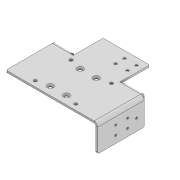
# Autodesk Inventor part: CCM_Mount_G
Saved by Autodesk Inventor 2020 (Build 240168000, 168)
## iProperties
Created: 2021-07-12
Part Number: CCM_Mount_G
Material: 一般
Document SubType Name: Sheet Metal
Designer: magnarecta
Density: 1 g/cm^3
Appearance: 既定
Sheet Metal Rule: Default
Author: magnarecta
Autodesk Inventor part; units mm, degrees
ref_plane "YZ Plane" through (0, 0, 0) normal (1, 0, 0) x (0, 1, 0)
ref_plane "XZ Plane" through (0, 0, 0) normal (0, 1, 0) x (-1, 0, 0)
ref_plane "XY Plane" through (0, 0, 0) normal (0, 0, 1) x (1, 0, 0)
sketch "スケッチ1" plane through (0, 0, 0) normal (0, 1, 0) x (-1, 0, 0)
  line L0 (-40, -39) -> (40, -39)
  line L1 (40, -39) -> (40, 39)
  line L2 (40, 39) -> (-40, 39)
  line L3 (-40, 39) -> (-40, -39)
  line L4 (-40, -39) -> (40, 39) construction
  line L5 (40, -39) -> (-40, 39) construction
  point P0 (0, 0)
  dimension "d0" = 80
  dimension "d1" = 78
  constraints: 12 end point, 2 midpoint, 2 parallel, 1 horizontal, 1 perpendicular
  measures "d0" distance of L0.start L0.end
  measures "d1" distance of L0.end L1.end
extrude "押し出し1" add sketch "スケッチ1" along normal blind 3
sketch "スケッチ2" plane through (0, 3, 0) normal (0, 1, 0) x (1, 0, 0)
  line L0 (34, 30) -> (-34, 30)
  line L1 (-34, 30) -> (-34, -30)
  line L2 (-34, -30) -> (34, -30)
  line L3 (34, -30) -> (34, 30)
  line L4 (34, 30) -> (-34, -30) construction
  line L5 (-34, 30) -> (34, -30) construction
  point P0 (0, 0)
  dimension "d4" = 68
  dimension "d5" = 60
  constraints: 12 end point, 2 midpoint, 2 parallel, 1 horizontal, 1 perpendicular
  measures "d4" distance of L2.end L1.end
  measures "d5" distance of L1.end L0.end
hole "穴1" at (-34, 3, 30) at (34, 3, 30) at (34, 3, -30) at (-34, 3, -30) direction (0, -1, 0) diameter 5.2 depth 8 tip angle 118
sketch "スケッチ3" plane through (0, 3, 0) normal (0, 1, 0) x (1, 0, 0)
  line L0 (13.5, 25) -> (-13.5, 25)
  line L1 (-13.5, 25) -> (-13.5, -25)
  line L2 (-13.5, -25) -> (13.5, -25)
  line L3 (13.5, -25) -> (13.5, 25)
  line L4 (13.5, 25) -> (-13.5, -25) construction
  line L5 (-13.5, 25) -> (13.5, -25) construction
  point P0 (0, 0)
  dimension "d13" = 27
  dimension "d14" = 50
  constraints: 12 end point, 4 coincident, 2 midpoint, 2 parallel, 1 horizontal, 1 perpendicular
  measures "d13" distance of L0.start L0.end
  measures "d14" distance of L0.end L1.end
hole "穴2" at (-13.5, 3, 25) at (13.5, 3, 25) at (13.5, 3, -25) at (-13.5, 3, -25) direction (0, -1, 0) diameter 5.3 depth 8 tip angle 118 countersink diameter 10 countersink angle 90
sketch "スケッチ5" plane through (0, 0, 0) normal (0, -1, 0) x (1, 0, 0)
  line L0 (74, 39) -> (-74, 39)
  line L1 (-74, 39) -> (-74, -39)
  line L2 (-74, -39) -> (74, -39)
  line L3 (74, -39) -> (74, 39)
  circle A0 centre (13.5, -25) radius 2.65 projected
  circle A1 centre (13.5, -25) radius 2.65 projected
  circle A2 centre (-13.5, 25) radius 2.65 projected
  circle A3 centre (13.5, 25) radius 2.65 projected
  circle A4 centre (-13.5, -25) radius 2.65 projected
  circle A5 centre (34, -30) radius 2.6 projected
  circle A6 centre (-34, 30) radius 2.6 projected
  circle A7 centre (34, 30) radius 2.6 projected
  circle A8 centre (-34, -30) radius 2.6 projected
  line L4 (-40, -39) -> (-40, 39) projected
  line L5 (40, -39) -> (-40, -39) projected
  line L6 (40, 39) -> (40, -39) projected
  line L7 (-40, 39) -> (40, 39) projected
  point P0 (0, 0)
  point P1 (-40, 39)
  dimension "d28" = 40
  dimension "d29" = 40
  constraints: 8 end point, 2 horizontal alignment, 2 parallel, 1 horizontal, 1 perpendicular
  measures "d28" distance from line of A5.centre L3
  measures "d29" distance from line of L1 A8.centre
extrude "押し出し3" add sketch "スケッチ5" against normal up to surface (3 mm away) contours L3 L2 L6 L0 | L4 L2 L1 L0
sketch "スケッチ6" plane through (0, 0, 0) normal (0, -1, 0) x (1, 0, 0)
  circle A0 centre (13.5, -25) radius 2.65 projected
  circle A1 centre (-13.5, 25) radius 2.65 projected
  circle A2 centre (13.5, 25) radius 2.65 projected
  circle A3 centre (-13.5, -25) radius 2.65 projected
  circle A4 centre (34, -30) radius 2.6 projected
  circle A5 centre (-34, 30) radius 2.6 projected
  circle A6 centre (34, 30) radius 2.6 projected
  circle A7 centre (-34, -30) radius 2.6 projected
  line L0 (-74, -39) -> (74, -39) projected
  line L1 (74, -39) -> (74, 39) projected
  line L2 (74, 39) -> (-74, 39) projected
  line L3 (-74, 39) -> (-74, -39) projected
  line L4 (74, -39) -> (44, -39)
  line L5 (44, -39) -> (44, -42)
  line L6 (44, -42) -> (74, -42)
  line L7 (74, -42) -> (74, -39)
  line L8 (-74, 39) -> (-74, -39) projected
  line L9 (-74, -39) -> (-44, -39)
  line L10 (-44, -39) -> (-44, -42)
  line L11 (-44, -42) -> (-74, -42)
  line L12 (-74, -42) -> (-74, -39)
  line L13 (44, -42) -> (-44, -42)
  line L14 (-44, -42) -> (-44, -39)
  line L15 (-44, -39) -> (44, -39)
  line L16 (44, -39) -> (44, -42)
  point P0 (0, 0)
  dimension "d33" = 30
  dimension "d34" = 30
  dimension "d49" = 3
  constraints: 24 end point, 6 parallel, 3 horizontal, 3 perpendicular, 1 horizontal alignment
  measures "d33" distance of L5.end L6.end
  measures "d34" distance of L10.end L11.end
  measures "d49" distance of L11.end L0.start
extrude "押し出し5" add sketch "スケッチ6" against normal up to surface (3 mm away) contours L0 L10 L11 L12 | L0 L7 L6 L5
sketch "スケッチ8" plane through (74, 0, -42) normal (0, 0, -1) x (-1, 0, 0)
  line L0 (30, 0) -> (0, 0)
  line L1 (0, 0) -> (0, -42)
  line L2 (0, -42) -> (30, -42)
  line L3 (30, -42) -> (30, 0)
  constraints: 6 end point, 1 horizontal, 1 perpendicular, 1 vertical
edge flange "フランジ2" height 45 angle 90 thickness 3 bend radius 3 thickness toward (0, 0, -1) relief straight relief width 3 relief depth 1.5 corner gap 3 corner form 0 edges at (59, 0, -42) (-59, 0, -42) wall of the first edge with corners at (44, 0, -42) (74, 0, -42) (74, -42, -42) (44, -42, -42)
bend "曲げ2"
corner "コーナー2"
fillet "フィレット3" radius 2 4 edges at (-74, -42, -43.5) (-44, -42, -43.5) (44, -42, -43.5) (74, -42, -43.5)
sketch "スケッチ9" plane through (-44, -3, -45) normal (0, 0, -1) x (-1, 0, 0)
  arc A0 (0, -37) -> (2, -39) centre (2, -37) ccw projected
  line L0 (28, -39) -> (2, -39) projected
  arc A1 (28, -39) -> (30, -37) centre (28, -37) ccw projected
  line L1 (30, 0) -> (30, -37) projected
  line L2 (30, 0) -> (0, 0) projected
  line L3 (0, -37) -> (0, 0) projected
  arc A2 (-118, -37) -> (-116, -39) centre (-116, -37) ccw projected
  line L4 (-90, -39) -> (-116, -39) projected
  arc A3 (-90, -39) -> (-88, -37) centre (-90, -37) ccw projected
  line L5 (-88, 0) -> (-88, -37) projected
  line L6 (-88, 0) -> (-118, 0) projected
  line L7 (-118, -37) -> (-118, 0) projected
  point P0 (-44, 3)
  point P1 (15, -29)
  point P2 (-103, -29)
  dimension "d63" = 15
  dimension "d64" = 15
  dimension "d65" = 10
  constraints: 1 horizontal alignment
  measures "d63" distance from line of point (15, -29) L1
  measures "d64" distance from line of L7 point (-103, -29)
  measures "d65" distance from line of L0 point (15, -29)
hole "穴3" at (-59, -32, -45) at (59, -32, -45) direction (0, 0, 1) diameter 6.2 depth 3 tip angle 118
sketch "スケッチ10" plane through (77, -3, 39) normal (1, 0, 0) x (0, 1, 0)
  line L0 (0, -78) -> (0, 0)
  line L1 (0, 0) -> (-39, 0)
  line L2 (-39, 0) -> (-39, -78)
  line L3 (-39, -78) -> (0, -78)
  constraints: 6 end point, 1 horizontal, 1 perpendicular, 1 vertical
edge flange "フランジ3" height 45 angle 90 thickness 3 bend radius 3 thickness toward (1, 0, 0) relief straight relief width 3 relief depth 1.5 edges at (74, 0, 0) wall of the first edge with corners at (77, -3, -39) (77, -3, 39) (77, -42, 39) (77, -42, -39)
bend "曲げ3"
corner "コーナー3"
fillet "フィレット4" radius 2 3 edges at (78.5, -42, -39) (78.5, -42, 39) (-74, 1.5, 39)
sketch "スケッチ11" plane through (80, -3, 39) normal (1, 0, 0) x (0, 0, -1)
  line L0 (30, -27) -> (50, -27)
  line L1 (50, -27) -> (50, -12)
  line L2 (50, -12) -> (30, -12)
  line L3 (30, -12) -> (30, -27)
  line L4 (76, -39) -> (2, -39) projected
  line L5 (0, -37) -> (0, 0) projected
  point P0 (39, 3)
  point P1 (50, -19.5)
  dimension "d84" = 15
  dimension "d85" = 19.5
  dimension "d86" = 50
  dimension "d87" = 20
  constraints: 8 end point, 2 parallel, 1 horizontal, 1 midpoint, 1 perpendicular
  measures "d84" distance of L0.end L1.end
  measures "d85" distance from line of point (50, -19.5) L4
  measures "d86" distance between parallel lines of L5 L1
  measures "d87" distance of L0.start L0.end
hole "穴4" at (80, -15, -11) at (80, -15, 9) at (80, -30, 9) at (80, -30, -11) direction (-1, 0, 0) diameter 3.242 end through all thread size "M4x0.7" class "6H" standard "ISO Metric profile"
sketch "スケッチ12" plane through (80, -3, 39) normal (1, 0, 0) x (0, 0, -1)
  circle A0 centre (30, -27) radius 1.621 projected
  circle A1 centre (50, -12) radius 1.621 projected
  circle A2 centre (30, -12) radius 1.621 projected
  circle A3 centre (50, -27) radius 1.621 projected
  arc A4 (0, -37) -> (2, -39) centre (2, -37) ccw projected
  line L0 (76, -39) -> (2, -39) projected
  arc A5 (76, -39) -> (78, -37) centre (76, -37) ccw projected
  line L1 (78, 0) -> (78, -37) projected
  line L2 (78, 0) -> (0, 0) projected
  line L3 (0, -37) -> (0, 0) projected
  point P0 (39, 3)
  point P1 (65, -19.5)
  dimension "d95" = 7.5
  dimension "d96" = 15
  measures "d95" vertical distance of A3.centre point (65, -19.5)
  measures "d96" horizontal distance of A3.centre point (65, -19.5)
hole "穴5" at (80, -22.5, -26) direction (-1, 0, 0) diameter 3.242 end through all thread size "M4x0.7" class "6H" standard "ISO Metric profile"
sketch "スケッチ13" plane through (0, 3, 0) normal (0, 1, 0) x (1, 0, 0)
  circle A0 centre (13.5, 25) radius 5 projected
  circle A1 centre (-13.5, -25) radius 5 projected
  circle A2 centre (13.5, -25) radius 5 projected
  circle A3 centre (-13.5, 25) radius 5 projected
  circle A4 centre (34, 30) radius 2.6 projected
  circle A5 centre (-34, -30) radius 2.6 projected
  circle A6 centre (34, -30) radius 2.6 projected
  circle A7 centre (-34, 30) radius 2.6 projected
  arc A8 (-74, -37) -> (-72, -39) centre (-72, -37) ccw projected
  line L0 (74, -39) -> (-72, -39) projected
  line L1 (74, 39) -> (74, -39) projected
  line L2 (44, 39) -> (74, 39) projected
  line L3 (-44, 39) -> (44, 39) projected
  line L4 (-74, 39) -> (-44, 39) projected
  line L5 (-74, -37) -> (-74, 39) projected
  line L6 (-44, 39) -> (44, 39) projected
  line L7 (-39, 39) -> (39, 39)
  line L8 (39, 39) -> (39, 89)
  line L9 (39, 89) -> (-39, 89)
  line L10 (-39, 89) -> (-39, 39)
  line L11 (44, 45) -> (44, 39) projected
  line L12 (-44, 39) -> (-44, 45) projected
  point P0 (0, 0)
  dimension "d104" = 50
  dimension "d105" = 5
  dimension "d106" = 5
  constraints: 8 end point, 2 parallel, 1 horizontal, 1 perpendicular, 1 point on line
  measures "d104" distance of L7.end L8.end
  measures "d105" distance between parallel lines of L11 L8
  measures "d106" distance between parallel lines of L10 L12
extrude "押し出し6" add sketch "スケッチ13" against normal up to surface (3 mm away) contours L10 L9 L8 L3
fillet "フィレット5" radius 2 2 edges at (39, 1.5, -89) (-39, 1.5, -89)
sketch "スケッチ14" plane through (0, 0, 0) normal (0, -1, 0) x (1, 0, 0)
  arc A0 (-39, -87) -> (-37, -89) centre (-37, -87) ccw projected
  line L0 (-37, -89) -> (37, -89) projected
  arc A1 (37, -89) -> (39, -87) centre (37, -87) ccw projected
  line L1 (39, -87) -> (39, -39) projected
  line L2 (39, -39) -> (44, -39) projected
  line L3 (44, -39) -> (74, -39) projected
  line L4 (74, -39) -> (74, 39) projected
  line L5 (74, 39) -> (-72, 39) projected
  arc A2 (-72, 39) -> (-74, 37) centre (-72, 37) ccw projected
  line L6 (-74, 37) -> (-74, -39) projected
  line L7 (-74, -39) -> (-44, -39) projected
  line L8 (-44, -39) -> (-39, -39) projected
  line L9 (-39, -39) -> (-39, -87) projected
  circle A3 centre (13.5, -25) radius 2.65 projected
  circle A4 centre (-13.5, 25) radius 2.65 projected
  circle A5 centre (13.5, 25) radius 2.65 projected
  circle A6 centre (-13.5, -25) radius 2.65 projected
  circle A7 centre (34, -30) radius 2.6 projected
  circle A8 centre (-34, 30) radius 2.6 projected
  circle A9 centre (34, 30) radius 2.6 projected
  circle A10 centre (-34, -30) radius 2.6 projected
  line L10 (9, -77) -> (29, -77)
  line L11 (29, -77) -> (29, -62)
  line L12 (29, -62) -> (9, -62)
  line L13 (9, -62) -> (9, -77)
  point P0 (0, 0)
  point P1 (29, -69.5)
  dimension "d110" = 15
  dimension "d111" = 19.5
  dimension "d112" = 10
  dimension "d113" = 20
  constraints: 8 end point, 2 parallel, 1 horizontal, 1 midpoint, 1 perpendicular
  measures "d110" distance of L10.end L11.end
  measures "d111" distance from line of point (29, -69.5) L0
  measures "d112" distance between parallel lines of L1 L11
  measures "d113" distance of L10.start L10.end
hole "穴6" at (9, 0, -62) at (9, 0, -77) at (29, 0, -77) at (29, 0, -62) direction (0, 1, 0) diameter 4.3 end through all countersink diameter 8 countersink angle 90
equation "\"d28\" = d29"
equation "\"d71\" = Thickness"
equation "\"d38\" = Thickness"
equation "\"d52\" = BendReliefWidth"
equation "\"d53\" = BendReliefDepth"
equation "\"d54\" = MinimumRemnant"
equation "\"d55\" = TransitionRadius"
equation "\"d58\" = BendRadius"
equation "\"d59\" = CornerReliefSize"
equation "\"d60\" = GapSize"
equation "\"d61\" = JacobiRadiusSize"
equation "\"d73\" = BendReliefWidth"
equation "\"d74\" = BendReliefDepth"
equation "\"d75\" = MinimumRemnant"
equation "\"d76\" = TransitionRadius"
equation "\"d79\" = BendRadius"
equation "\"d80\" = CornerReliefSize"
equation "\"d81\" = GapSize"
equation "\"d82\" = JacobiRadiusSize"
equation "\"BendRadius\" = Thickness"
equation "\"BendReliefWidth\" = Thickness"
equation "\"BendReliefDepth\" = 0.5 * Thickness"
equation "\"CornerReliefSize\" = 4 * Thickness"
equation "\"MinimumRemnant\" = 2 * Thickness"
equation "\"TransitionRadius\" = BendRadius"
equation "\"JacobiRadiusSize\" = Thickness"
equation "\"GapSize\" = Thickness"
equation "\"Thickness\" = 3"
